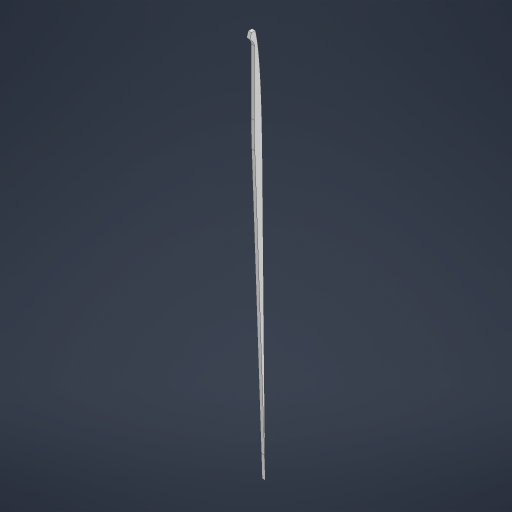
# Autodesk Inventor part: standoff
Saved by Autodesk Inventor 2024 (Build 280153000, 153)
## iProperties
Created: 2022-03-24
Part Number: standoff
Material: Generic
Document SubType Name: Modeling
Designer: kardo
Density: 1 g/cm^3
Appearance: Default
Mass: 4.32367 g
Surface Area: 51.1498 cm^2
Volume: 4.32367 cm^3
Author: kardo
Autodesk Inventor part; units mm, degrees
ref_plane "YZ Plane" through (0, 0, 0) normal (1, 0, 0) x (0, 1, 0)
ref_plane "XZ Plane" through (0, 0, 0) normal (0, 1, 0) x (-1, 0, 0)
ref_plane "XY Plane" through (0, 0, 0) normal (0, 0, 1) x (1, 0, 0)
derived "parameters_frame.ipt"
derived "surface_body.ipt"
sketch "sk_rail_bottom_standoff" plane through (34.32, 0, 0) normal (1, 0, 0) x (0, 1, 0)
  line L0 (-345, 16.32) -> (-262.2001, 18.586)
  arc A0 (-262.2001, 18.586) -> (-241.5001, 19.2432) centre (-326.8578, 2381.2399) ccw
  line L1 (36.465, 28.832) -> (112.2, 28.832)
  arc A1 (36.465, 28.832) -> (11.22, 28.376) centre (36.465, -670.197) ccw
  line L2 (-241.5001, 19.2432) -> (11.22, 28.376)
  line L3 (-465, 0) -> (375, 0) construction
  line L4 (11.22, 28.376) -> (11.22, 0) construction
  line L5 (-241.5001, 19.2432) -> (-241.5001, 0) construction
  point P0 (0, 0)
  point P1 (-241.5001, 19.1524)
  point P2 (11.22, 28.832)
sketch "sk_rail_standoff_standoff" plane through (34.32, 0, 0) normal (1, 0, 0) x (0, 1, 0)
  line L0 (0, 21.3303) -> (92.004, 22.2293) construction
  line L1 (92.004, 22.2293) -> (112.2, 28.832) construction
  line L2 (0, 21.3303) -> (-241.5001, 18.9703)
  line L3 (-262.2001, 18.586) -> (-345, 16.32)
  arc A0 (-241.5001, 18.9703) -> (-262.2001, 18.586) centre (-229.9974, -1158.1286) ccw
  line L4 (-465, 0) -> (375, 0) construction
  line L5 (-241.5001, 18.9703) -> (-241.5001, 0) construction
  spline S0 degree 2 poles (0, 21.3303) (92.004, 22.2293) (112.2, 28.832) knots 1 1 1 2 2 2
  point P0 (0, 0)
  point P1 (-241.5001, 19.1524)
ref_plane "plane_standoff_right" through (34.32, 0, 0) normal (1, 0, 0) x (0, 1, 0)
ref_plane "plane_nose" through (0, 112.2, 0) normal (0, 1, 0) x (-1, 0, 0)
ref_plane "plane_tail_1" through (0, -114.9999, 0) normal (0, 1, 0) x (-1, 0, 0)
sketch "sk_rail_top_tunnel" plane through (81.12, 0, 0) normal (1, 0, 0) x (0, 1, 0)
  line L0 (255, 107.6209) -> (255, -224.5198) construction
  line L1 (0, 107.6209) -> (0, -224.5198) construction
  line L2 (-345, 107.6209) -> (-345, -224.5198) construction
  line L3 (-345, 0) -> (0, 0) construction
  line L4 (-172.5, 48.8998) -> (-172.5, 0) construction
  line L5 (0, 52.89) -> (37.026, 52.89) construction
  line L6 (37.026, 52.89) -> (80.784, 47.0555) construction
  line L7 (80.784, 47.0555) -> (112.2, 37.536) construction
  line L8 (112.2, 107.6209) -> (112.2, -224.5198) construction
  line L9 (0, 52.89) -> (255, 52.89) construction
  line L10 (-469.9275, 0) -> (379.2584, 0) construction
  spline S0 degree 3 poles (0, 52.89) (92.8353, 52.89) (195.0311, 49.5089) (255, 36.448) knots 0 0 0 0 1 1 1 1
  spline S1 degree 3 poles (0, 52.89) (37.026, 52.89) (80.784, 47.0555) (112.2, 37.536) knots 1 1 1 1 2 2 2 2
  spline S2 degree 4 poles (-345, 37.3935) (-258.8686, 45.1235) (-172.5923, 49.7074) (-86.3167, 52.89) (0, 52.89) knots 0 0 0 0 0 1 1 1 1 1
  point P0 (153, 48.7795)
  point P1 (112.2, 28.832)
  point P2 (-230.0001, 45.8224)
  point P3 (-114.9999, 50.9907)
sketch "sk_base" plane through (34.32, 0, 0) normal (1, 0, 0) x (0, 1, 0)
  arc A0 (-241.5001, 18.9703) -> (-262.2001, 18.586) centre (-229.9974, -1158.1286) ccw construction
  arc A1 (-262.2001, 18.586) -> (-241.5001, 19.2432) centre (-326.8578, 2381.2399) ccw construction
  line L0 (-241.5001, 19.2432) -> (11.22, 28.376) construction
  line L1 (0, 21.3303) -> (-241.5001, 18.9703) construction
  spline S0 degree 2 poles (0, 21.3303) (92.004, 22.2293) (112.2, 28.832) knots 1 1 1 2 2 2 construction
  line L2 (36.465, 28.832) -> (112.2, 28.832) construction
  arc A2 (36.465, 28.832) -> (11.22, 28.376) centre (36.465, -670.197) ccw construction
  line L3 (-0.0078, 22.1302) -> (-241.5079, 19.7703)
  arc A3 (-241.5079, 19.7703) -> (-262.2001, 19.3863) centre (-229.9974, -1158.1286) ccw
  arc A4 (-262.2001, 19.3863) -> (-241.529, 20.0427) centre (-326.8578, 2381.2399) ccw
  line L4 (-241.529, 20.0427) -> (11.1911, 29.1755)
  arc A5 (36.465, 29.632) -> (11.1911, 29.1755) centre (36.465, -670.197) ccw
  line L5 (36.465, 29.632) -> (109.2, 29.632)
  line L6 (-262.2001, 18.586) -> (-262.2001, 19.3863) construction
  line L7 (109.2, 28.8048) -> (109.2, 29.632)
  line L8 (109.2, 36.036) -> (109.2, 29.632)
  line L9 (112.2, 3089.1136) -> (112.2, -1866.0023) construction
  line L10 (-114.9999, 3089.1136) -> (-114.9999, -1866.0023) construction
  spline S1 degree 3 poles (0, 52.89) (37.026, 52.89) (80.784, 47.0555) (112.2, 37.536) knots 1 1 1 1 2 2 2 2 construction
  line L11 (109.2, 36.036) -> (112.2, 36.036) construction
  spline S2 degree 3 poles (109.2, 36.036) (104.3654, 36.036) (101.9121, 29.632) (97.0775, 29.632) knots 0 0 0 0 1 1 1 1
  spline S3 degree 5 poles (109.2, 28.8047) (107.6034, 28.4007) (105.9915, 28.0566) (104.3743, 27.7461) (99.4475, 26.8968) (94.4884, 26.2578) (91.1573, 25.8839) (83.3512, 25.1123) (75.5281, 24.5312) (71.0451, 24.2412) (60.9319, 23.667) (50.8112, 23.2411) (45.1777, 23.0388) (32.7621, 22.6576) (20.3433, 22.3976) (13.5599, 22.2846) (6.7761, 22.1965) (-0.0078, 22.1302) knots 0 0 0 0 0 0 0.075161 0.075161 0.075161 0.228117 0.228117 0.228117 0.433128 0.433128 0.433128 0.690387 0.690387 0.690387 1 1 1 1 1 1
  point P0 (0, 0)
  dimension "d5" = 0.8
  dimension "d4" = 0.8
  dimension "d7" = 3
  dimension "d8" = 1.5
  dimension "d9" = 72.735
  dimension "d10" = 12.1225
  constraints: 14 end point, 6 point on circle, 3 centre point, 3 vertical, 2 parallel, 2 point on line, 1 horizontal, 1 perpendicular, 9 other
  measures "d4" distance between parallel lines of L0 L4
  measures "d7" distance between parallel lines of L9 L7
  measures "d8" distance from line of point (112.2, 37.536) L11
  measures "d9" distance of L5.start L5.end
  measures "d10" distance from line of L8 point (97.077, 29.632)
extrude "thicken" add sketch "sk_base" against normal blind 3
sketch "sk_liner_pad" plane through (34.32, 0, 0) normal (1, 0, 0) x (0, 1, 0)
  spline S0 degree 3 poles (0, 52.89) (37.026, 52.89) (80.784, 47.0555) (112.2, 37.536) knots 1 1 1 1 2 2 2 2 projected
  line L0 (112.2, 37.536) -> (112.2, 31.536)
  line L1 (112.2, 107.6209) -> (112.2, -224.5198) construction
  line L2 (0, 52.89) -> (0, 46.89)
  spline S1 degree 3 poles (0, 46.89) (37.9228, 46.89) (75.8479, 42.5512) (112.2, 31.536) knots 0 0 0 0 1 1 1 1
  line L3 (0, 52.89) -> (-10, 52.89) construction
  line L4 (0, 46.89) -> (-10, 46.89) construction
  line L5 (112.2, 37.536) -> (121.7703, 34.6361) construction
  line L6 (112.2, 31.536) -> (121.7703, 28.6361) construction
  point P0 (0, 0)
  dimension "d11" = 6
  dimension "d12" = 10
  dimension "d13" = 10
  constraints: 12 end point, 6 parallel, 2 horizontal, 1 point on line, 4 other
  measures "d11" distance of L0.start L0.end
  measures "d12" distance of L2.start L3.end
  measures "d13" distance of L0.start L5.end
extrude "liner_pad" cut sketch "sk_liner_pad" along normal through all both and the other way through all
equation "\"d4\" = shell_thickness"
equation "\"d7\" = bulkhead_thickness"
equation "\"d8\" = cowl_shell_thickness"
equation "\"d10\" = 0.166667 * d9"
equation "\"d2\" = bulkhead_thickness"
equation "\"d11\" = cowl_sealing_thickness + cowl_shell_thickness + cowl_liner_thickness"
equation "\"shell_thickness\" = 0.8"
equation "\"bulkhead_thickness\" = 3"
equation "\"cowl_sealing_thickness\" = 3"
equation "\"cowl_shell_thickness\" = 1.5"
equation "\"cowl_liner_thickness\" = 1.5"
body "Solid1"
